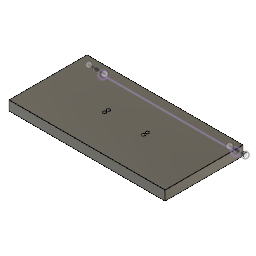
Semana4_Desafio6 (tampa) v2 (Autodesk Fusion 360 design; units mm, degrees)
Autodesk Fusion 360 part; units mm, degrees
sketch "Sketch1" plane through (0, 0, 0) normal (0, 0, 1) x (1, 0, 0)
  line L0 (200, -100) -> (-200, -100)
  line L1 (-200, -100) -> (-200, 100)
  line L2 (-200, 100) -> (200, 100)
  line L3 (200, 100) -> (200, -100)
  line L4 (200, -100) -> (-200, 100) construction
  line L5 (-200, -100) -> (200, 100) construction
  line L6 (195, -95) -> (-195, -95)
  line L7 (-195, -95) -> (-195, 95)
  line L8 (-195, 95) -> (195, 95)
  line L9 (195, 95) -> (195, -95)
  line L10 (195, -95) -> (-195, 95) construction
  line L11 (-195, -95) -> (195, 95) construction
  dimension "d1" = 400
  dimension "d2" = 200
  dimension "d3" = 390
  dimension "d4" = 190
  constraint horizontal L0
  constraint perpendicular L0 L1
  constraint parallel L0 L2
  constraint parallel L1 L3
  constraint coincident L4 origin
  constraint coincident L5 origin
  constraint horizontal L6
  constraint perpendicular L6 L7
  constraint parallel L6 L8
  constraint parallel L7 L9
  constraint coincident L10 origin
  constraint coincident L11 origin
  measures "d1" distance of L1.end L2.end
  measures "d2" distance of L0.end L1.end
  measures "d3" distance of L7.end L8.end
  measures "d4" distance of L6.end L7.end
extrude "Extrude1" add sketch "Sketch1" along normal blind 25
sketch "Sketch2" plane through (0, 0, 25) normal (0, 0, 1) x (-1, 0, 0)
  line L0 (195, -95) -> (-195, -95)
  line L1 (-195, -95) -> (-195, 95)
  line L2 (-195, 95) -> (195, 95)
  line L3 (195, 95) -> (195, -95)
  line L4 (-200, -100) -> (200, -100)
  line L5 (200, -100) -> (200, 100)
  line L6 (200, 100) -> (-200, 100)
  line L7 (-200, 100) -> (-200, -100)
  line L8 (-200, 100) -> (200, 100)
  line L9 (200, 100) -> (200, -100)
  line L10 (200, -100) -> (-200, -100)
  line L11 (-200, -100) -> (-200, 100)
  line L12 (-200, 100) -> (200, -100) construction
  line L13 (200, 100) -> (-200, -100) construction
  constraint horizontal L8
  constraint perpendicular L8 L9
  constraint parallel L8 L10
  constraint parallel L9 L11
  constraint coincident L6.end L7.start
  constraint coincident L12 origin
  constraint coincident L13 origin
extrude "Extrude2" add sketch "Sketch2" against normal blind 10 contours L0 L1 L2 L3
sketch "Sketch3" plane through (0, 0, 0) normal (0, 0, -1) x (1, 0, 0)
  line L0 (195, -95) -> (-195, -95)
  line L1 (-195, -95) -> (-195, 95)
  line L2 (-195, 95) -> (195, 95)
  line L3 (195, 95) -> (195, -95)
  line L4 (-200, -100) -> (200, -100)
  line L5 (200, -100) -> (200, 100)
  line L6 (200, 100) -> (-200, 100)
  line L7 (-200, 100) -> (-200, -100)
  line L8 (200, -100) -> (200, -97.5)
  line L9 (200, -97.5) -> (180, -97.5)
  line L10 (180, -97.5) -> (180, -100)
  line L11 (200, -100) -> (180, -100)
  line L12 (-180, -100) -> (-180, -97.5)
  line L13 (-180, -97.5) -> (-160, -97.5)
  line L14 (-160, -97.5) -> (-160, -100)
  line L15 (-160, -100) -> (-180, -100)
  dimension "d9" = 2.5
  dimension "d11" = 20
  dimension "d12" = 2.5
  dimension "d13" = 20
  dimension "d14" = 20
  constraint coincident L4 L5.start
  constraint perpendicular L0 L8
  constraint perpendicular L8 L9
  constraint coincident L4 L10.end
  constraint perpendicular L4 L10
  constraint collinear L5 L8
  constraint coincident L4 L12.start
  constraint perpendicular L4 L12
  constraint perpendicular L12 L13
  constraint coincident L4 L14.end
  constraint perpendicular L4 L14
  measures "d9" distance of L4.end L8.end
  measures "d11" distance of L8 L10
  measures "d12" distance of L12.start L12.end
  measures "d13" distance of L12.end L13.end
  measures "d14" distance of L7 L12
extrude "Extrude3" cut sketch "Sketch3" against normal blind 7.5 contours L4 L12 L13 L14 L15 | L4 L5 L8 L9 L10 L11
sketch "Sketch4" plane through (0, 0, 0) normal (0, 0, 1) x (1, 0, 0)
  line L0 (200, 105) -> (160, 105)
  line L1 (-160.0025, 105) -> (-199.9975, 105)
  line L2 (-160, 100) -> (180, 100)
  point P0 (-180, 105)
  point P1 (180, 105)
  dimension "d17" = 5
  constraint horizontal L0
  constraint horizontal L1
  constraint midpoint L1 P0
  constraint midpoint L0 P1
  constraint horizontal P0 P1
  measures "d17" distance of L0 L2
pipe "Pipe1" add diameter 10 path "Sketch4" along L0
pipe "Pipe2" add diameter 10 path "Sketch4" along L1
fillet "Fillet1" radius 0.5 1 edges at (200, 109.6616, -1.8081)
fillet "Fillet2" radius 0.5 1 edges at (-160.0025, 109.6616, -1.8081)
sketch "Sketch7" plane through (0, 0, 15) normal (0, 0, -1) x (1, 0, 0)
  line L0 (195, 95) -> (-195, 95)
  line L1 (-195, 95) -> (-195, -95)
  line L2 (-195, -95) -> (195, -95)
  line L3 (195, -95) -> (195, 95)
  line L4 (-55, 10) -> (-55, -10) construction
  line L5 (-55, -10) -> (-45, -10) construction
  line L6 (-45, -10) -> (-45, 10) construction
  line L7 (-45, 10) -> (-55, 10) construction
  line L8 (55, 0) -> (55, 10) construction
  line L9 (55, 10) -> (45, 10) construction
  line L10 (45, 10) -> (45, -10) construction
  line L11 (45, -10) -> (55, -10) construction
  line L12 (55, -10) -> (55, 0) construction
  circle A0 centre (50, 5) radius 4
  circle A1 centre (50, -5) radius 4
  circle A2 centre (-50, 5) radius 4
  circle A3 centre (-50, -5) radius 4
  dimension "d64" = 8
  dimension "d65" = 8
  dimension "d66" = 8
  dimension "d67" = 8
  constraint vertical L4
  constraint perpendicular L4 L5
  constraint perpendicular L5 L6
  constraint perpendicular L6 L7
  constraint vertical L8
  constraint perpendicular L8 L9
  constraint perpendicular L9 L10
  constraint perpendicular L10 L11
  constraint perpendicular L11 L12
  measures "d64" diameter of A0
  measures "d65" diameter of A1
  measures "d66" diameter of A2
  measures "d67" diameter of A3
extrude "Extrude5" cut sketch "Sketch7" against normal blind 10 contours A0 | A1 | A2 | A3
